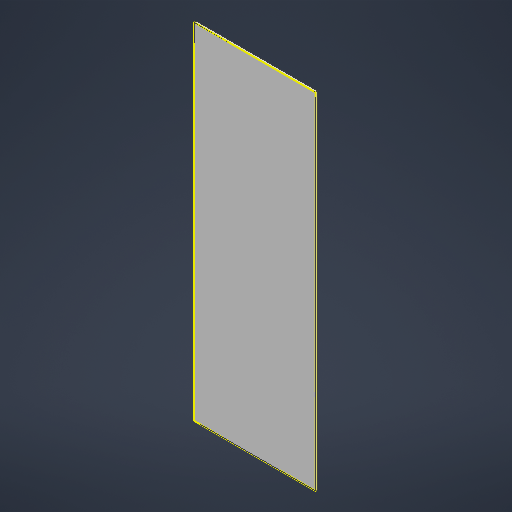
# Autodesk Inventor part: TAMPA
Saved by Autodesk Inventor 2026 (Build 300175050, 175E)
## iProperties
Created: 2025-08-11
Part Number: TAMPA
Material: Genérico
Document SubType Name: Modeling
Designer: EspacoMaker
Density: 1 g/cm^3
Appearance: Padrão
Author: EspacoMaker
Autodesk Inventor part; units mm, degrees
ref_plane "YZ Plane" through (0, 0, 0) normal (1, 0, 0) x (0, 1, 0)
ref_plane "XZ Plane" through (0, 0, 0) normal (0, 1, 0) x (-1, 0, 0)
ref_plane "XY Plane" through (0, 0, 0) normal (0, 0, 1) x (1, 0, 0)
sketch "Esboço1" plane through (0, 0, 0) normal (0, 0, 1) x (1, 0, 0)
  line L0 (-53.8, 153) -> (53.8, 153)
  line L1 (53.8, 153) -> (53.8, -153)
  line L2 (53.8, -153) -> (-53.8, -153)
  line L3 (-53.8, -153) -> (-53.8, 153)
  line L4 (-53.8, 153) -> (53.8, -153) construction
  line L5 (53.8, 153) -> (-53.8, -153) construction
  point P0 (0, 0)
  dimension "d0" = 306
  dimension "d1" = 107.6
  constraints: 12 end point, 2 midpoint, 2 parallel, 1 horizontal, 1 perpendicular
  measures "d0" distance of L0.end L1.end
  measures "d1" distance of L0.start L0.end
extrude "Extrusão1" add sketch "Esboço1" along normal blind 2
sketch "Esboço2" plane through (0, 0, 2) normal (0, 0, 1) x (1, 0, 0)
  line L0 (-53.8, -153) -> (53.8, -153) projected
  line L1 (53.8, -153) -> (53.8, 153) projected
  line L2 (53.8, 153) -> (-53.8, 153) projected
  line L3 (-53.8, 153) -> (-53.8, -153) projected
